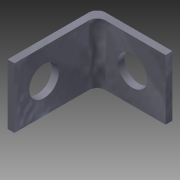
# Autodesk Inventor part: LBracket
Saved by Autodesk Inventor 2016 (Build 200138000, 138)
## iProperties
Created: 2015-04-30
Part Number: LBracket
Material: Generic
Document SubType Name: Modeling
Designer: Admin
Density: 1 g/cm^3
Appearance: Weld - Stainless Steel
Author: Admin
Autodesk Inventor part; units mm, degrees
ref_plane "YZ Plane" through (0, 0, 0) normal (1, 0, 0) x (0, 1, 0)
ref_plane "XZ Plane" through (0, 0, 0) normal (0, 1, 0) x (-1, 0, 0)
ref_plane "XY Plane" through (0, 0, 0) normal (0, 0, 1) x (1, 0, 0)
sketch "Sketch1" plane through (0, 0, 0) normal (0, 0, 1) x (1, 0, 0)
  line L0 (-4.455, 5.305) -> (4.455, 5.305)
  line L1 (4.455, 5.305) -> (4.455, -5.305)
  line L2 (4.455, -5.305) -> (-4.455, -5.305)
  line L3 (-4.455, -5.305) -> (-4.455, 5.305)
  line L4 (-6.237, 0) -> (6.237, 0) projected
  line L5 (0, -7.427) -> (0, 7.427) projected
  point P0 (0, 0)
  dimension "d0" = 8.91
  dimension "d1" = 10.61
  dimension "d2" = 4.455
  dimension "d3" = 5.305
  constraints: 8 end point, 2 parallel, 1 horizontal, 1 perpendicular
  measures "d0" distance of L1.end L2.end
  measures "d1" distance of L0.end L1.end
  measures "d2" distance between parallel lines of L5 L1
  measures "d3" distance between parallel lines of L4 L0
extrude "BraketBase" add sketch "Sketch1" along normal blind 7.13
sketch "Sketch2" plane through (0, 0, 7.13) normal (0, 0, 1) x (1, 0, 0)
  line L0 (4.455, 5.305) -> (-4.455, 5.305) projected
  line L1 (-4.455, 5.305) -> (-4.455, -5.305) projected
  line L2 (-4.455, -5.305) -> (4.455, -5.305) projected
  line L3 (4.455, -5.305) -> (4.455, 5.305) projected
  line L4 (-3.635, 4.485) -> (4.455, 4.485)
  line L5 (-3.635, 4.485) -> (-3.635, -5.305)
  line L6 (-4.455, -5.305) -> (4.455, -5.305) projected
  line L7 (-3.635, 4.485) -> (4.455, 4.485)
  line L8 (4.455, 4.485) -> (4.455, -5.305)
  line L9 (4.455, -5.305) -> (-3.635, -5.305)
  line L10 (-3.635, -5.305) -> (-3.635, 4.485)
  point P0 (0, 0)
  dimension "d6" = 0.82
  dimension "d7" = 0.82
  constraints: 12 end point, 2 horizontal, 2 parallel, 2 perpendicular, 2 point on line
  measures "d6" distance between parallel lines of L0 L4
  measures "d7" distance from line of L5.end L1
extrude "BraketCut" cut sketch "Sketch2" against normal blind 7.13 contours L3 L2 L5 L4
sketch "Sketch3" plane through (-4.455, 5.305, 0) normal (0, 1, 0) x (1, 0, 0)
  line L0 (0, 0) -> (8.91, 0) projected
  line L1 (0, 0) -> (0, -7.13) projected
  line L2 (8.91, -7.13) -> (0, -7.13) projected
  line L3 (8.91, 0) -> (8.91, -7.13) projected
  circle A0 centre (5, -3.565) radius 1.75
  point P0 (4.455, 0)
  dimension "d10" = 3.5
  dimension "d11" = 5
  dimension "d12" = 3.565
  constraints: 1 centre point
  measures "d10" diameter of A0
  measures "d11" distance from line of L1 A0.centre
  measures "d12" distance from line of A0.centre L2
hole "ShortHole" at (0.545, 5.305, 3.565) direction (0, -1, 0) diameter 3.5 end through all
sketch "Sketch4" plane through (-3.635, -5.305, 7.13) normal (1, 0, 0) x (0, 0, -1)
  line L0 (0, 0) -> (0, 9.79) projected
  line L1 (7.13, 0) -> (0, 0) projected
  line L2 (7.13, 9.79) -> (7.13, 0) projected
  line L3 (0, 9.79) -> (7.13, 9.79) projected
  circle A0 centre (3.565, 3.5) radius 1.75
  point P0 (7.13, 5.305)
  dimension "d20" = 3.5
  dimension "d21" = 3.5
  dimension "d22" = 3.565
  constraints: 1 centre point
  measures "d20" diameter of A0
  measures "d21" distance from line of L1 A0.centre
  measures "d22" distance from line of L2 A0.centre
hole "LongHole" at (-3.635, -1.805, 3.565) direction (-1, 0, 0) diameter 3.5 end through all
fillet "Fillet1" radius 1 2 edges at (-4.455, 5.305, 3.565) (-3.635, 4.485, 3.565)
equation "\"d2\" = 0.5 * d0"
equation "\"d3\" = 0.5 * d1"
equation "\"d7\" = d6"
body "Solid1"
